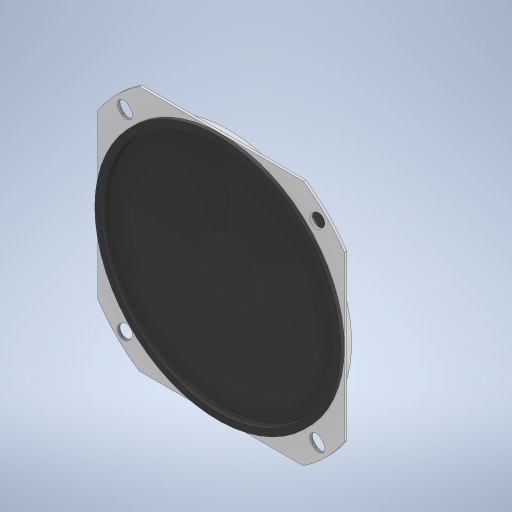
# Autodesk Inventor part: 스피커
Saved by Autodesk Inventor 2023.1 (Build 271208000, 208)
## iProperties
Created: 2022-08-14
Part Number: 스피커
Material: 일반
Document SubType Name: Modeling
Designer: fly01
Density: 1 g/cm^3
Appearance: 기본값
Author: fly01
Autodesk Inventor part; units mm, degrees
ref_plane "YZ Plane" through (0, 0, 0) normal (1, 0, 0) x (0, 1, 0)
ref_plane "XZ Plane" through (0, 0, 0) normal (0, 1, 0) x (-1, 0, 0)
ref_plane "XY Plane" through (0, 0, 0) normal (0, 0, 1) x (1, 0, 0)
sketch "스케치1" plane through (0, 0, 0) normal (0, 0, 1) x (1, 0, 0)
  circle A0 centre (0, 0) radius 46.25
  line L0 (-38.5, 38.5) -> (38.5, 38.5)
  line L1 (38.5, 38.5) -> (38.5, -38.5)
  line L2 (38.5, -38.5) -> (-38.5, -38.5)
  line L3 (-38.5, -38.5) -> (-38.5, 38.5)
  line L4 (-38.5, 38.5) -> (38.5, -38.5) construction
  line L5 (38.5, 38.5) -> (-38.5, -38.5) construction
  point P0 (-38.5, 25.6284)
  point P1 (-38.5, -25.6284)
  point P2 (-25.6284, -38.5)
  point P3 (25.6284, -38.5)
  point P4 (38.5, -25.6284)
  point P5 (38.5, 25.6284)
  point P6 (25.6284, 38.5)
  point P7 (-25.6284, 38.5)
  dimension "d0" = 92.5
  dimension "d1" = 77
  dimension "d2" = 77
  constraints: 12 end point, 2 midpoint, 2 parallel, 1 centre point, 1 coincident, 1 horizontal, 1 perpendicular
  measures "d0" diameter of A0
  measures "d1" distance of L0.start L0.end
  measures "d2" distance of L0.end L1.end
extrude "돌출1" add sketch "스케치1" along normal blind 0.75 contours L1 A0 L2 L3 L0
sketch "스케치2" plane through (0, 0, 0) normal (0, 1, 0) x (-1, 0, 0)
  line L0 (25.6284, 0.75) -> (-25.6284, 0.75) projected
  line L1 (0, 0.75) -> (0, -28.2062)
  line L2 (38.5, 0) -> (38.5, -1.5)
  line L3 (38.5, -1.5) -> (35, -1.5)
  line L4 (35, -1.5) -> (35, -3.59)
  line L5 (35, -3.59) -> (0, -3.59)
  line L6 (38.5, 0) -> (25.6284, 0) projected
  line L7 (30, -3.59) -> (17.5, -9.59)
  line L8 (17.5, -9.59) -> (15, -11.99)
  line L9 (15, -11.99) -> (15, -21.99)
  line L10 (15, -21.99) -> (0, -21.99)
  line L11 (-25.6284, 0) -> (25.6284, 0) projected
  point P0 (0, 0)
  point P1 (0, 0)
  dimension "d5" = 1.5
  dimension "d6" = 2.09
  dimension "d7" = 77
  dimension "d8" = 70
  dimension "d9" = 60
  dimension "d10" = 35
  dimension "d11" = 30
  dimension "d12" = 6
  dimension "d13" = 2.4
  dimension "d14" = 10
  constraints: 18 end point, 4 perpendicular, 4 point on line, 3 vertical, 1 midpoint
  measures "d5" distance of L2.start L2.end
  measures "d6" distance of L3.end L4.end
  measures "d7" diameter of L2.start L1
  measures "d8" diameter of L4 L1
  measures "d9" diameter of L7.start L1
  measures "d10" diameter of L7.end L1
  measures "d11" diameter of L8.end L1
  measures "d12" vertical distance of L7.start L7.end
  measures "d13" vertical distance of L8.end L7.end
  measures "d14" distance of L8.end L9.end
revolve "회전1" add sketch "스케치2" angle 360 about axis through (0, 0, 0.75) along (0, 0, -1)
sketch "스케치3" plane through (0, 0, 0) normal (0, 1, 0) x (-1, 0, 0)
  line L0 (38.5, 0) -> (38.5, 0.75) projected
  line L1 (38.5, 0.75) -> (38.5, 1.75)
  line L2 (38.5, 1.75) -> (36.3, 1.75)
  line L3 (36.3, 1.75) -> (36.3, 0.75)
  line L4 (38.5, 0.75) -> (25.6284, 0.75) projected
  line L5 (9.1955, -2.25) -> (0, -2.25)
  line L6 (-35, -1.5) -> (35, -1.5) projected
  line L7 (0, -2.25) -> (0, 0.75)
  line L8 (25.6284, 0.75) -> (-25.6284, 0.75) projected
  line L9 (36.3, 0.75) -> (0, 0.75)
  line L10 (0, 0) -> (-25.6284, 0) projected
  line L11 (36.3, 0.75) -> (36.3, -0.45)
  line L12 (36.3, -0.45) -> (9.1955, -2.25)
  point P0 (20.489, -1.5)
  point P1 (0, -1.5)
  dimension "d16" = 1
  dimension "d17" = 2.2
  dimension "d18" = 1.2
  dimension "d19" = 3
  constraints: 16 end point, 2 parallel, 2 perpendicular, 2 point on line, 1 midpoint, 1 vertical
  measures "d16" distance of L2.end L3.end
  measures "d17" distance of L1.end L2.end
  measures "d18" distance of L3.end L11.end
  measures "d19" distance of L5.end L7.end
revolve "회전2" add sketch "스케치3" angle 360 about axis through (0, 0, -2.25) along (0, 0, 1) contours L4 L3 L2 L1
revolve "회전3" cut sketch "스케치3" angle 360 about axis through (0, 0, -2.25) along (0, 0, 1) contours L11 L12 L6 L7 L8 L4 | L12 L5 L7 L6
sketch "스케치4" plane through (0, 0, 0.75) normal (0, 0, 1) x (1, 0, 0)
  circle A0 centre (0, 0) radius 42 construction
  line L0 (0, 0) -> (0, 16.8085)
  line L1 (0, 0) -> (-29.6985, 29.6985) construction
  line L2 (-29.6985, 29.6985) -> (-30.4056, 30.4056) construction
  line L3 (-28.2843, 31.1127) -> (-28.9914, 31.8198)
  line L4 (-31.8198, 28.9914) -> (-31.1127, 28.2843)
  arc A1 (-31.1127, 28.2843) -> (-28.2843, 31.1127) centre (-29.6985, 29.6985) ccw
  arc A2 (-28.9914, 31.8198) -> (-31.8198, 28.9914) centre (-30.4056, 30.4056) ccw
  point P0 (-30.052, 30.052)
  dimension "d22" = 84
  dimension "d23" = 45
  dimension "d24" = 1
  dimension "d25" = 4
  constraints: 12 end point, 4 point on circle, 4 tangent, 2 centre point, 1 coincident, 1 midpoint, 1 parallel, 1 vertical, 3 other
  measures "d23" angle of L0 L1
  measures "d24" distance of L1.end L2.end
  measures "d25" diameter of A2
extrude "돌출2" cut sketch "스케치4" against normal blind 0.75
pattern_circular "원형 패턴1" count 4 over 360 about axis through (0, 0, 1.25) along (0, 0, 1) of "돌출2"
